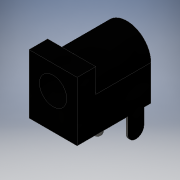
# Autodesk Inventor part: 5mm_BarrelJack
Saved by Autodesk Inventor 2016 (Build 200138000, 138)
## iProperties
Created: 2016-09-23
Part Number: 5mm_BarrelJack
Material: Generic
Document SubType Name: Modeling
Designer: jfixelle
Density: 1 g/cm^3
Appearance: Black
Author: jfixelle
Autodesk Inventor part; units mm, degrees
ref_plane "YZ Plane" through (0, 0, 0) normal (1, 0, 0) x (0, 1, 0)
ref_plane "XZ Plane" through (0, 0, 0) normal (0, 1, 0) x (-1, 0, 0)
ref_plane "XY Plane" through (0, 0, 0) normal (0, 0, 1) x (1, 0, 0)
sketch "Sketch1" plane through (0, 0, 0) normal (0, 0, 1) x (1, 0, 0)
  line L0 (-4.4, 10.85) -> (4.4, 10.85)
  line L1 (4.4, 10.85) -> (4.4, 0)
  line L2 (4.4, 0) -> (-4.4, 0)
  line L3 (-4.4, 0) -> (-4.4, 10.85)
  point P0 (0, 0)
  dimension "d0" = 8.8
  dimension "d1" = 4.4
  dimension "d2" = 0
  dimension "d3" = 10.85
  constraints: 8 end point, 2 parallel, 1 horizontal, 1 perpendicular
  measures "d0" distance of L0.start L0.end
  measures "d1" distance from line of point (0, 0) L1
  measures "d2" distance from line of point (0, 0) L2
  measures "d3" distance between parallel lines of L2 L0
extrude "Extrusion1" add sketch "Sketch1" against normal blind 3.4
sketch "Sketch2" plane through (0, 0, -3.4) normal (0, 0, -1) x (-1, 0, 0)
  line L0 (-4.4, 10.85) -> (-4.4, 0) projected
  line L1 (-4.4, 6.45) -> (-4.4, 5.425)
  line L2 (4.4, 10.85) -> (-4.4, 10.85) projected
  line L3 (4.4, 0) -> (4.4, 10.85) projected
  line L4 (4.4, 6.45) -> (4.4, 4.887)
  arc A0 (4.4, 6.45) -> (-4.4, 6.45) centre (0, 6.45) ccw
  line L5 (-4.4, 0) -> (4.4, 0) projected
  line L6 (-4.4, 5.425) -> (-4.4, 0)
  line L7 (-4.4, 0) -> (4.4, 0)
  line L8 (4.4, 0) -> (4.4, 4.887)
  point P0 (0, 0)
  constraints: 10 end point, 3 tangent, 2 perpendicular, 2 point on circle, 1 centre point, 1 collinear, 1 midpoint, 1 point on line
extrude "Extrusion2" add sketch "Sketch2" along normal blind 10.1 contours A0 L3 L5 L0
sketch "Sketch3" plane through (0, 0, 0) normal (0, 0, 1) x (1, 0, 0)
  circle A0 centre (0, 6.5) radius 2.5
  line L0 (-4.4, 10.85) -> (4.4, 10.85) projected
  point P0 (0, 0)
  dimension "d8" = 4.35
  dimension "d9" = 5
  constraints: 1 centre point
  measures "d8" distance from line of L0 A0.centre
  measures "d9" diameter of A0
extrude "Extrusion3" cut sketch "Sketch3" against normal blind 8
sketch "Sketch4" plane through (-4.4, 0, 0) normal (0, -1, 0) x (1, 0, 0)
  line L0 (8.8, -3.4) -> (8.8, -13.5) projected
  line L1 (8.8, -9.6102) -> (8.8, -6.6102)
  line L2 (0, -13.5) -> (8.8, -13.5) projected
  line L3 (5.9, -13.5) -> (2.9, -13.5)
  line L4 (2.9, -13.5) -> (2.9, -13.2)
  line L5 (2.9, -13.2) -> (5.9, -13.2)
  line L6 (5.9, -13.2) -> (5.9, -13.5)
  line L7 (8.5, -12.24) -> (8.8, -12.24)
  line L8 (8.8, -12.24) -> (8.8, -9.24)
  line L9 (8.8, -9.24) -> (8.5, -9.24)
  line L10 (8.5, -9.24) -> (8.5, -12.24)
  line L11 (2.9, -7.49) -> (5.9, -7.49)
  line L12 (5.9, -7.49) -> (5.9, -7.74)
  line L13 (5.9, -7.74) -> (2.9, -7.74)
  line L14 (2.9, -7.74) -> (2.9, -7.49)
  line L15 (8.8, 0) -> (0, 0) projected
  point P0 (4.4, 0)
  dimension "d12" = 3
  dimension "d14" = 3
  dimension "d15" = 1.5
  dimension "d16" = 3
  dimension "d17" = 1.5
  dimension "d18" = 0.3
  dimension "d19" = 0.25
  dimension "d20" = 0.3
  dimension "d22" = 9.24
  dimension "d24" = 7.49
  dimension "d28" = 0
  constraints: 26 end point, 6 parallel, 3 horizontal, 3 perpendicular, 2 point on line
  measures "d12" distance of L7.end L8.end
  measures "d14" distance of L4.end L5.end
  measures "d15" distance from line of L6 point (4.4, 0)
  measures "d16" distance of L12.end L13.end
  measures "d17" distance from line of point (4.4, 0) L12
  measures "d18" distance of L8.end L9.end
  measures "d19" distance of L13.end L11.start
  measures "d20" distance of L3.end L4.end
  measures "d22" distance between parallel lines of L9 L15
  measures "d24" distance between parallel lines of L11 L15
  measures "d28" distance between parallel lines of L0 L8
extrude "Extrusion4" add sketch "Sketch4" along normal blind 4.3
fillet "Fillet1" radius 1.5 6 edges at (4.25, -4.3, -9.24) (4.25, -4.3, -12.24) (-1.5, -4.3, -7.615) (1.5, -4.3, -7.615) (-1.5, -4.3, -13.35) (1.5, -4.3, -13.35)
body "Solid1"
